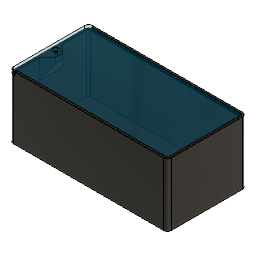
box-generator (Autodesk Fusion 360 design; units mm, degrees)
Autodesk Fusion 360 part; units mm, degrees
sketch "SketchBottom" plane through (0, 0, 0) normal (0, 0, 1) x (1, 0, 0)
  line L0 (95, 50) -> (-95, 50)
  line L1 (-100, 45) -> (-100, -45)
  line L2 (-95, -50) -> (95, -50)
  line L3 (100, -45) -> (100, 45)
  line L4 (100, 50) -> (-100, -50) construction
  line L5 (-100, 50) -> (100, -50) construction
  arc A0 (-100, -45) -> (-95, -50) centre (-95, -45) ccw
  arc A1 (-95, 50) -> (-100, 45) centre (-95, 45) ccw
  arc A2 (100, 45) -> (95, 50) centre (95, 45) ccw
  arc A3 (95, -50) -> (100, -45) centre (95, -45) ccw
  line L6 (-97.5, 45) -> (-97.5, -45)
  arc A4 (-97.5, -45) -> (-95, -47.5) centre (-95, -45) ccw
  line L7 (-95, -47.5) -> (95, -47.5)
  arc A5 (95, -47.5) -> (97.5, -45) centre (95, -45) ccw
  line L8 (97.5, -45) -> (97.5, 45)
  arc A6 (97.5, 45) -> (95, 47.5) centre (95, 45) ccw
  line L9 (95, 47.5) -> (-95, 47.5)
  arc A7 (-95, 47.5) -> (-97.5, 45) centre (-95, 45) ccw
  dimension "d7" = 200
  dimension "d8" = 100
  dimension "d9" = 5
  constraint horizontal L0
  constraint perpendicular L0 L1
  constraint parallel L0 L2
  constraint parallel L1 L3
  constraint coincident L4 origin
  constraint coincident L5 origin
  constraint coincident L4.end L2
  constraint coincident L4.end L1
  constraint tangent L2 A0
  constraint tangent L1 A0
  constraint coincident L5.start L1
  constraint coincident L5.start L0
  constraint tangent L1 A1
  constraint tangent L0 A1
  constraint equal A0 A1
  constraint coincident L4.start L0
  constraint coincident L4.start L3
  constraint tangent L0 A2
  constraint tangent L3 A2
  constraint equal A0 A2
  constraint coincident L5.end L3
  constraint coincident L5.end L2
  constraint tangent L3 A3
  constraint tangent L2 A3
  constraint equal A0 A3
  measures "d7" distance of L4.end L5.end
  measures "d8" distance of L5.start L4.end
  measures "d9" radius of A0
extrude "ExtrudeWall" add sketch "SketchBottom" along normal blind 76 makes body 1
extrude "ExtrudeBottom" add sketch "SketchBottom" along normal blind 3 contours L6 A4 L7 A5 L8 A6 L9 A7 bodies 1
sketch "SketchLidWall" plane through (0, 0, 76) normal (0, 0, 1) x (-1, 0, 0)
  arc A0 (95, -47.5) -> (97.5, -45) centre (95, -45) ccw
  line L0 (95, -47.5) -> (-95, -47.5)
  arc A1 (-97.5, -45) -> (-95, -47.5) centre (-95, -45) ccw
  line L1 (-97.5, -45) -> (-97.5, 45)
  arc A2 (-95, 47.5) -> (-97.5, 45) centre (-95, 45) ccw
  line L2 (-95, 47.5) -> (95, 47.5)
  arc A3 (97.5, 45) -> (95, 47.5) centre (95, 45) ccw
  line L3 (97.5, 45) -> (97.5, -45)
  arc A4 (-95, 50) -> (-100, 45) centre (-95, 45) ccw
  line L4 (-100, 45) -> (-100, -45)
  arc A5 (-100, -45) -> (-95, -50) centre (-95, -45) ccw
  line L5 (-95, -50) -> (95, -50)
  arc A6 (95, -50) -> (100, -45) centre (95, -45) ccw
  line L6 (100, -45) -> (100, 45)
  arc A7 (100, 45) -> (95, 50) centre (95, 45) ccw
  line L7 (95, 50) -> (-95, 50)
  line L8 (98.5, -45) -> (98.5, 45)
  arc A8 (98.5, 45) -> (95, 48.5) centre (95, 45) ccw
  line L9 (95, 48.5) -> (-95, 48.5)
  arc A9 (-95, 48.5) -> (-98.5, 45) centre (-95, 45) ccw
  line L10 (-98.5, 45) -> (-98.5, -45)
  arc A10 (-98.5, -45) -> (-95, -48.5) centre (-95, -45) ccw
  line L11 (-95, -48.5) -> (95, -48.5)
  arc A11 (95, -48.5) -> (98.5, -45) centre (95, -45) ccw
extrude "ExtrudeLidWall" add sketch "SketchLidWall" along normal blind 2.5 contours A4 L4 A5 L5 A6 L6 A7 L7 bodies 1
sketch "SketchLidWallTop" plane through (0, 0, 78.5) normal (0, 0, 1) x (-1, 0, 0)
  arc A0 (95, -48.5) -> (98.5, -45) centre (95, -45) ccw
  line L0 (95, -48.5) -> (-95, -48.5)
  arc A1 (-98.5, -45) -> (-95, -48.5) centre (-95, -45) ccw
  line L1 (-98.5, -45) -> (-98.5, 45)
  arc A2 (-95, 48.5) -> (-98.5, 45) centre (-95, 45) ccw
  line L2 (-95, 48.5) -> (95, 48.5)
  arc A3 (98.5, 45) -> (95, 48.5) centre (95, 45) ccw
  line L3 (98.5, 45) -> (98.5, -45)
  line L4 (95, 50) -> (-95, 50)
  arc A4 (-95, 50) -> (-100, 45) centre (-95, 45) ccw
  line L5 (-100, 45) -> (-100, -45)
  arc A5 (-100, -45) -> (-95, -50) centre (-95, -45) ccw
  line L6 (-95, -50) -> (95, -50)
  arc A6 (95, -50) -> (100, -45) centre (95, -45) ccw
  line L7 (100, -45) -> (100, 45)
  arc A7 (100, 45) -> (95, 50) centre (95, 45) ccw
  line L8 (97.5, -45) -> (97.5, 45)
  arc A8 (97.5, 45) -> (95, 47.5) centre (95, 45) ccw
  line L9 (95, 47.5) -> (-95, 47.5)
  arc A9 (-95, 47.5) -> (-97.5, 45) centre (-95, 45) ccw
  line L10 (-97.5, 45) -> (-97.5, -45)
  arc A10 (-97.5, -45) -> (-95, -47.5) centre (-95, -45) ccw
  line L11 (-95, -47.5) -> (95, -47.5)
  arc A11 (95, -47.5) -> (97.5, -45) centre (95, -45) ccw
extrude "ExtrudeLidWallTop" add sketch "SketchLidWallTop" along normal blind 1.5 contours A0 L0 A1 L1 A2 L2 A3 L3 | L4 A4 L5 A5 L6 A6 L7 A7 bodies 1
sketch "SketchLidCutOut" plane through (0, 0, 80) normal (0, 0, 1) x (-1, 0, 0)
  arc A0 (95, -47.5) -> (97.5, -45) centre (95, -45) ccw
  line L0 (95, -47.5) -> (-95, -47.5)
  arc A1 (-97.5, -45) -> (-95, -47.5) centre (-95, -45) ccw
  line L1 (-97.5, -45) -> (-97.5, 45)
  arc A2 (-95, 47.5) -> (-97.5, 45) centre (-95, 45) ccw
  line L2 (-95, 47.5) -> (95, 47.5)
  arc A3 (97.5, 45) -> (95, 47.5) centre (95, 45) ccw
  line L3 (97.5, 45) -> (97.5, -45)
  arc A4 (100, 45) -> (95, 50) centre (95, 45) ccw
  line L4 (95, 50) -> (-95, 50)
  arc A5 (-95, 50) -> (-100, 45) centre (-95, 45) ccw
  line L5 (-100, 45) -> (-100, -45)
  arc A6 (-100, -45) -> (-95, -50) centre (-95, -45) ccw
  line L6 (-95, -50) -> (95, -50)
  arc A7 (95, -50) -> (100, -45) centre (95, -45) ccw
  line L7 (100, -45) -> (100, 45)
  line L8 (100, 0) -> (93, 0) construction
  line L9 (93, 50) -> (93, -50)
  dimension "d26" = 7
  dimension "d27" = 100
  constraint midpoint L7 L8.start
  constraint perpendicular L3 L8
  constraint midpoint L8.end L9
  constraint perpendicular L6 L9
  measures "d26" distance of L8.start L8.end
  measures "d27" distance of L9.start L9.end
extrude "ExtrudeLidCutOut" cut sketch "SketchLidCutOut" against normal blind 4 contours A0 L0 L2 A3 L3 A4 L4 L6 A7 L7 L9 bodies 1
chamfer "ChamberBoxLid" distance 1 distance2 1.5 5 edges at (1, 48.5, 78.5) (97.4749, 47.4749, 78.5) (98.5, 0, 78.5) (97.4749, -47.4749, 78.5) (1, -48.5, 78.5) measured on face at (32.3333, 47.8333, 78.5) measured on face at (32.3333, 47.8333, 78.5) measured on face at (32.3333, 47.8333, 78.5) measured on face at (32.3333, 47.8333, 78.5) measured on face at (32.3333, 47.8333, 78.5) on bodies 1
sketch "SketchLid" plane through (0, 0, 76) normal (0, 0, 1) x (-1, 0, 0)
  line L0 (93, 48.5) -> (-95, 48.5)
  arc A0 (-95, 48.5) -> (-98.5, 45) centre (-95, 45) ccw
  line L1 (-98.5, 45) -> (-98.5, -45)
  arc A1 (-98.5, -45) -> (-95, -48.5) centre (-95, -45) ccw
  line L2 (-95, -48.5) -> (93, -48.5)
  line L3 (93, -48.5) -> (93, -50)
  line L4 (93, -50) -> (95, -50)
  arc A2 (95, -50) -> (100, -45) centre (95, -45) ccw
  line L5 (100, -45) -> (100, 45)
  arc A3 (100, 45) -> (95, 50) centre (95, 45) ccw
  line L6 (95, 50) -> (93, 50)
  line L7 (93, 50) -> (93, 48.5)
  line L8 (-95, 47.5) -> (95, 47.5)
  arc A4 (97.5, 45) -> (95, 47.5) centre (95, 45) ccw
  line L9 (97.5, 45) -> (97.5, -45)
  arc A5 (95, -47.5) -> (97.5, -45) centre (95, -45) ccw
  line L10 (95, -47.5) -> (-95, -47.5)
  arc A6 (-97.5, -45) -> (-95, -47.5) centre (-95, -45) ccw
  line L11 (-97.5, -45) -> (-97.5, 45)
  arc A7 (-95, 47.5) -> (-97.5, 45) centre (-95, 45) ccw
  line L12 (99.85, -45) -> (99.85, 45)
  arc A8 (99.85, 45) -> (95, 49.85) centre (95, 45) ccw
  line L13 (95, 49.85) -> (93.15, 49.85)
  line L14 (93.15, 49.85) -> (93.15, 48.35)
  line L15 (93.15, 48.35) -> (-95, 48.35)
  arc A9 (-95, 48.35) -> (-98.35, 45) centre (-95, 45) ccw
  line L16 (-98.35, 45) -> (-98.35, -45)
  arc A10 (-98.35, -45) -> (-95, -48.35) centre (-95, -45) ccw
  line L17 (-95, -48.35) -> (93.15, -48.35)
  line L18 (93.15, -48.35) -> (93.15, -49.85)
  line L19 (93.15, -49.85) -> (95, -49.85)
  arc A11 (95, -49.85) -> (99.85, -45) centre (95, -45) ccw
  line L20 (100, 0) -> (93.15, 0) construction
  line L21 (93.15, -50) -> (93.15, 50)
  dimension "d42" = 6.85
  dimension "d43" = 100
  constraint midpoint L5 L20.start
  constraint perpendicular L5 L20
  constraint midpoint L20.end L21
  constraint perpendicular L20 L21
  measures "d42" distance of L20.start L20.end
  measures "d43" distance of L21.start L21.end
extrude "ExtrudeLid" add sketch "SketchLid" along normal blind 2.5 separate body contours L4 A2 L5 A3 L6 L12 A8 L13 L19 A11 L21 | L8 A4 L9 A5 L10 L12 A8 L13 L14 L18 L19 A11 L21 | L8 L10 A6 L11 A7 L15 A9 L16 A10 L17 L21 | L8 L10 A6 L11 A7 L21 | L8 A4 L9 A5 L10 L21 makes body 2
chamfer "ChamberLid" distance 1 distance2 1.5 5 edges at (0.925, 48.35, 78.5) (0.925, -48.35, 78.5) (97.3688, -47.3688, 78.5) (98.35, 0, 78.5) (97.3688, 47.3688, 78.5) measured on face at (32.2833, -16.1167, 78.5) measured on face at (32.2833, -16.1167, 78.5) measured on face at (32.2833, -16.1167, 78.5) measured on face at (32.2833, -16.1167, 78.5) measured on face at (32.2833, -16.1167, 78.5) on bodies 2
extrude "ExtrudeLidTop" add 1 faces at (32.2833, -15.7833, 78.5) along direction (0, 0, 1) blind 1.5 on bodies 2 bodies 2
sketch "SketchBlockThread" plane through (-97.5, 0, 0) normal (1, 0, 0) x (0, 1, 0)
  line L0 (-45, 3) -> (45, 3)
  line L1 (45, 3) -> (45, 76)
  line L2 (45, 76) -> (-45, 76)
  line L3 (-45, 76) -> (-45, 3)
  line L4 (0, 76) -> (-4.4, 76) construction
  line L5 (-4.4, 76) -> (4.4, 76)
  line L6 (4.4, 76) -> (4.4, 69.3)
  line L7 (4.4, 69.3) -> (-4.4, 69.3)
  line L8 (-4.4, 69.3) -> (-4.4, 76)
  dimension "d54" = 4.4
  dimension "d56" = 8.8
  dimension "d57" = 6.7
  constraint midpoint L2 L4.start
  constraint parallel L2 L4
  constraint horizontal L5
  constraint vertical L6
  constraint horizontal L7
  constraint vertical L8
  measures "d54" distance of L4.start L4.end
  measures "d56" distance of L4.end L5.end
  measures "d57" distance of L4.end L7.end
extrude "ExtrudeBlockThread" add sketch "SketchBlockThread" along normal blind 10.3 contours L2 L5 L6 L7 L8 bodies 1
chamfer "ChamberBlockThread" distance 18.9 distance2 10.3 1 edges at (-97.5, 0, 69.3) measured on face at (-97.5, 1.4667, 25.1) on bodies 1
sketch "SketchThreadHole" plane through (0, 0, 76) normal (0, 0, 1) x (-1, 0, 0)
  line L0 (93, 48.5) -> (-95, 48.5)
  arc A0 (-95, 48.5) -> (-98.5, 45) centre (-95, 45) ccw
  line L1 (-98.5, 45) -> (-98.5, -45)
  arc A1 (-98.5, -45) -> (-95, -48.5) centre (-95, -45) ccw
  line L2 (-95, -48.5) -> (93, -48.5)
  line L3 (93, -48.5) -> (93, -50)
  line L4 (93, -50) -> (95, -50)
  arc A2 (95, -50) -> (100, -45) centre (95, -45) ccw
  line L5 (100, -45) -> (100, 45)
  arc A3 (100, 45) -> (95, 50) centre (95, 45) ccw
  line L6 (95, 50) -> (93, 50)
  line L7 (93, 50) -> (93, 48.5)
  line L8 (-95, 47.5) -> (95, 47.5)
  arc A4 (97.5, 45) -> (95, 47.5) centre (95, 45) ccw
  line L9 (97.5, 45) -> (97.5, 4.4)
  line L10 (97.5, 4.4) -> (87.2, 4.4)
  line L11 (87.2, 4.4) -> (87.2, -4.4)
  line L12 (87.2, -4.4) -> (97.5, -4.4)
  line L13 (97.5, -4.4) -> (97.5, -45)
  arc A5 (95, -47.5) -> (97.5, -45) centre (95, -45) ccw
  line L14 (95, -47.5) -> (-95, -47.5)
  arc A6 (-97.5, -45) -> (-95, -47.5) centre (-95, -45) ccw
  line L15 (-97.5, -45) -> (-97.5, 45)
  arc A7 (-95, 47.5) -> (-97.5, 45) centre (-95, 45) ccw
  line L16 (87.2, 0) -> (91.12, 0) construction
  circle A8 centre (91.12, 0) radius 2
  circle A9 centre (91.12, 0) radius 1.6
  dimension "d60" = 3.92
  dimension "d61" = 4
  dimension "d67" = 3.2
  constraint midpoint L11 L16.start
  constraint perpendicular L11 L16
  constraint coincident L16.end A8.centre
  constraint concentric A8 A9
  measures "d60" distance of L16.start L16.end
  measures "d61" diameter of A8
  measures "d67" diameter of A9
extrude "ExtrudeThredHole" cut sketch "SketchThreadHole" against normal blind 6.7 contours A8 | A9 bodies 1
extrude "ExtrudeLidSrewHole" cut sketch "SketchThreadHole" along normal blind 9 contours A9 bodies 2
chamfer "ChamberScrewHole" distance 2 distance2 2 1 edges at (-89.6283, -0.5786, 80) measured on face at (33.4884, 0.0726, 80) on bodies 2
chamfer "ChamberScrewBlow" distance 10.3 distance2 10.3 2 edges at (-97.5, -4.4, 63.2) (-97.5, 4.4, 63.2) measured on face at (-97.5, 1.4667, 18.8013) measured on face at (-97.5, 1.4667, 18.8013) on bodies 1
chamfer "ChamberAllCorners" distance 0.2 distance2 0.2 8 edges at (100, 0, 0) (98.5355, 48.5355, 0) (0, 50, 0) (-98.5355, 48.5355, 0) (-100, 0, 0) (-98.5355, -48.5355, 0) (0, -50, 0) (98.5355, -48.5355, 0) measured on face at (100, -15, 53.3333) measured on face at (95.9463, 49.9096, 26.6667) measured on face at (32.3333, 50, 52) measured on face at (-98.6187, 48.4504, 25.3333) measured on face at (-100, 15, 25.3333) measured on face at (-95.9463, -49.9096, 50.6667) measured on face at (32.3333, -50, 52) measured on face at (98.9303, -48.0908, 26.6667) on bodies 1 2
chamfer "ChamberAllCorners" distance 0.2 distance2 0.2 5 edges at (100, 0, 80) (98.5355, -48.5355, 80) (1, -50, 80) (1, 50, 80) (98.5355, 48.5355, 80) measured on face at (32.3333, 48.3333, 80) measured on face at (32.3333, 48.3333, 80) measured on face at (32.3333, 48.3333, 80) measured on face at (32.3333, 48.3333, 80) measured on face at (32.3333, 48.3333, 80) on bodies 1 2
chamfer "ChamberAllCorners" distance 0.2 distance2 0.2 5 edges at (-100, 0, 80) (-98.5355, 48.5355, 80) (-94.075, 50, 80) (-94.075, -50, 80) (-98.5355, -48.5355, 80) measured on face at (34.16, 0, 80) measured on face at (34.16, 0, 80) measured on face at (34.16, 0, 80) measured on face at (34.16, 0, 80) measured on face at (34.16, 0, 80) on bodies 1 2
chamfer "ChamberAllCorners" distance 0.2 distance2 0.2 12 edges at (-97.5, 29.85, 76) (-96.7678, 46.7678, 76) (0, 47.5, 76) (96.7678, 46.7678, 76) (97.5, 0, 76) (96.7678, -46.7678, 76) (0, -47.5, 76) (-96.7678, -46.7678, 76) (-97.5, -29.85, 76) (-92.35, 9.55, 76) (-87.2, 0, 76) (-92.35, -9.55, 76) measured on face at (-96.04, 0, 76) measured on face at (-96.04, 0, 76) measured on face at (-96.04, 0, 76) measured on face at (-96.04, 0, 76) measured on face at (-96.04, 0, 76) measured on face at (-96.04, 0, 76) measured on face at (-96.04, 0, 76) measured on face at (-96.04, 0, 76) measured on face at (-96.04, 0, 76) measured on face at (-94.0674, 11.2653, 65.2346) measured on face at (-87.2, -1.4667, 73.7667) measured on face at (-94.0674, -11.2653, 65.2346) on bodies 1 2
copy_body "Body->Comp1" bodies 2 removing the originals makes body 3 in component "LID"
copy_body "Body->Comp2" bodies 1 removing the originals makes body 4 in component "BOX"
component "LID" placed x (1, 0, 0) y (0, 1, 0) z (0, 0, 1) at (0, 0, 0)
component "BOX" placed x (1, 0, 0) y (0, 1, 0) z (0, 0, 1) at (0, 0, 0)
equation "box_width = 100 mm"
equation "box_length = 200 mm"
equation "box_hight = 80 mm"
equation "wall_thickness = 2.5 mm"
equation "bottom_thickness = 3 mm"
equation "corner_radius = 5 mm"
equation "d7 = box_length"
equation "d8 = box_width"
equation "d9 = corner_radius"
equation "d10 = -wall_thickness"
equation "d11 = box_hight - LidWallTopHight - LidWallHight"
equation "d13 = bottom_thickness"
equation "d20 = -LidWallThickness"
equation "d21 = LidWallHight"
equation "d23 = -wall_thickness"
equation "d24 = LidWallTopHight"
equation "d26 = LidCutOut"
equation "d27 = box_width"
equation "d28 = -LidWallHight - LidWallTopHight"
equation "LidWallHight = 2.5 mm"
equation "LidWallTopHight = 1.5 mm"
equation "LidCutOut = 7 mm"
equation "LidWallThickness = 1.5 mm"
equation "d34 = wall_thickness - LidWallThickness"
equation "d35 = LidWallHight - 1 mm"
equation "LidOffset = 0.15 mm"
equation "d41 = -LidOffset"
equation "d42 = LidCutOut - LidOffset"
equation "d43 = box_width"
equation "d44 = LidWallHight"
equation "d46 = wall_thickness - LidWallThickness"
equation "d47 = LidWallHight - 1 mm"
equation "d48 = LidWallTopHight"
equation "HoleThread = 4 mm"
equation "MinSideWithHoleThread = 1.6 mm"
equation "ThreadDepth = 6.7 mm"
equation "d54 = ( MinSideWithHoleThread * 1.5 ) + ( HoleThread / 2 )"
equation "d56 = d54 * 2"
equation "d57 = ThreadDepth"
equation "d58 = ( ( MinSideWithHoleThread * 1.5 * 2 ) - wall_thickness ) + ( HoleThread ) + 4 mm"
equation "d60 = ( MinSideWithHoleThread * 1.2 ) + ( HoleThread / 2 )"
equation "d61 = HoleThread"
equation "d62 = ( ( ( MinSideWithHoleThread * 1.5 * 2 ) - wall_thickness ) + ( HoleThread ) ) * 3"
equation "d63 = ( ( MinSideWithHoleThread * 1.5 * 2 ) - wall_thickness ) + ( HoleThread ) + 4 mm"
equation "d64 = -ThreadDepth"
equation "ScrewDiameter = 3 mm"
equation "d67 = ScrewDiameter + 0.2 mm"
equation "d68 = LidWallHight + LidWallThickness + 5 mm"
equation "d80 = ( ( MinSideWithHoleThread * 1.5 * 2 ) - wall_thickness ) + ( HoleThread ) + 4 mm"
equation "d81 = ( ( MinSideWithHoleThread * 1.5 * 2 ) - wall_thickness ) + ( HoleThread ) + 4 mm"
named bodies: "BOX", "LID"
